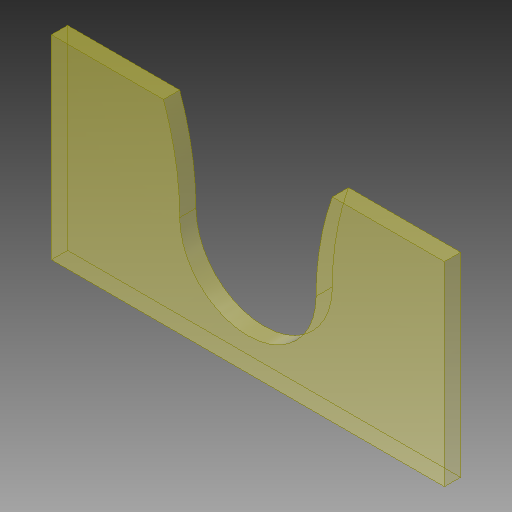
# Autodesk Inventor part: surround_front back
Saved by Autodesk Inventor 2018.1 (Build 221171000, 171)
## iProperties
Created: 2017-07-30
Part Number: surround_front back
Material: PVC-Piping
Document SubType Name: Modeling
Designer: Tom
Density: 1.4 g/cm^3
Appearance: Clear - Yellow
Mass: 27.823 g
Surface Area: 116.531 cm^2
Volume: 19.8735 cm^3
Author: Tom
Autodesk Inventor part; units mm, degrees
ref_plane "YZ Plane" through (0, 0, 0) normal (1, 0, 0) x (0, 1, 0)
ref_plane "XZ Plane" through (0, 0, 0) normal (0, 1, 0) x (-1, 0, 0)
ref_plane "XY Plane" through (0, 0, 0) normal (0, 0, 1) x (1, 0, 0)
sketch "Sketch1" plane through (0, 0, 0) normal (0, 0, 1) x (1, 0, 0)
  line L0 (0, 0) -> (121, 0)
  line L1 (121, 0) -> (121, 60)
  line L2 (121, 60) -> (0, 60)
  line L3 (0, 60) -> (0, 0)
  dimension "d0" = 121
  dimension "d1" = 60
  constraints: 8 end point, 2 parallel, 1 horizontal, 1 perpendicular
  measures "d0" distance of L2.end L1.end
  measures "d1" distance of L1.end L0.end
extrude "Extrusion1" add sketch "Sketch1" along normal blind 5
sketch "Sketch2" plane through (0, 0, 5) normal (0, 0, 1) x (1, 0, 0)
  circle A0 centre (60.5, 45.5856) radius 9.2358
  line L0 (121, 60) -> (0, 60) construction
  line L1 (60.5, 60) -> (60.5, 0) construction
  line L2 (0, 0) -> (121, 0) construction
  constraints: 2 end point, 2 midpoint, 1 centre point, 1 point on line
extrude "Extrusion2" cut sketch "Sketch2" against normal blind 5
sketch "Sketch4" plane through (0, 0, 5) normal (0, 0, 1) x (1, 0, 0)
  circle A0 centre (60.5, 31) radius 16 construction
  line L0 (0, 0) -> (121, 0) construction
  line L1 (60.5, 0) -> (60.5, 60) construction
  line L2 (60.5, 60) -> (34.5, 60) construction
  arc A1 (39.5, 31) -> (81.5, 31) centre (60.5, 31) ccw
  line L3 (60.5, 31) -> (81.5, 31) construction
  line L4 (60.5, 31) -> (39.5, 31) construction
  line L5 (60.5, 60) -> (86.5, 60) construction
  line L6 (121, 60) -> (0, 60) construction
  line L7 (34.5, 60) -> (86.5, 60)
  arc A2 (39.5, 31) -> (34.5, 60) centre (-47.1, 31) ccw
  arc A3 (86.5, 60) -> (81.5, 31) centre (168.1, 31) ccw
  dimension "d28" = 26
  dimension "d30" = 21
  dimension "d33" = 32
  dimension "d34" = 180
  dimension "d35" = 90
  dimension "d36" = 26
  dimension "d39" = 0
  constraints: 12 end point, 6 point on circle, 3 centre point, 2 tangent, 1 coincident, 1 collinear, 1 midpoint, 1 point on line
  measures "d28" distance of L1.end L2.end
  measures "d30" radius of A1
  measures "d33" diameter of A0
  measures "d34" angle of L3 L4
  measures "d35" angle of L1 L4
  measures "d36" distance of L1.end L5.end
  measures "d39" distance from line of L6 L1.end
extrude "Extrusion5" cut sketch "Sketch4" against normal blind 5
equation "\"d0\" = tankw + 2 * slack + 2 * surroundt + 2 * pvct"
equation "\"d1\" = surroundh"
equation "\"d2\" = surroundt"
equation "\"d4\" = surroundt"
equation "\"d30\" = 0.5 * diasurroundhole"
equation "\"d37\" = surroundt"
equation "\"lcsd\" = 19.05"
equation "\"lcwd1\" = 25"
equation "\"lcwd2\" = 34"
equation "\"lch1\" = 39"
equation "\"lcwd3\" = 43"
equation "\"dia1\" = 6"
equation "\"td\" = 18"
equation "\"bhh\" = 6"
equation "\"sw\" = 25"
equation "\"sh\" = 31"
equation "\"spacert\" = 2"
equation "\"pvct\" = 5"
equation "\"tankl\" = 379"
equation "\"dia4\" = 11"
equation "\"dia3\" = 8"
equation "\"play\" = 9"
equation "\"holeh\" = 26"
equation "\"surroundh\" = 60"
equation "\"slack\" = 0.5"
equation "\"surroundt\" = 5"
equation "\"play2\" = 3"
equation "\"diaair\" = 32"
equation "\"diacucl\" = 32"
equation "\"diawater\" = 25"
equation "\"diaph\" = 32"
equation "\"diaoverflow\" = 25"
equation "\"diasurroundhole\" = 42"
equation "\"diagrate\" = 12"
equation "\"gratespacing\" = 12.02082"
equation "\"bottomdist\" = 9.6355"
equation "\"sidedist\" = 13.9375"
equation "\"diahcl\" = 32"
equation "\"bracketwtop\" = 6"
equation "\"bracketwbottom\" = 6"
equation "\"nett\" = 1"
equation "\"nethole\" = 16"
equation "\"nettop\" = 7"
equation "\"netside\" = 3.5"
equation "\"netholespacing\" = 2"
equation "\"diaetape\" = 32"
equation "\"tankw\" = 100"
body "Solid1"
